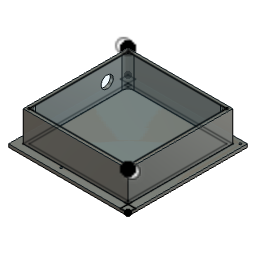
battery enclosure v1 (Autodesk Fusion 360 design; units mm, degrees)
Autodesk Fusion 360 part; units mm, degrees
sketch "Sketch1" plane through (0, 0, 0) normal (0, 1, 0) x (1, 0, 0)
  line L0 (0, 0) -> (196, 0)
  line L1 (196, 0) -> (196, 196)
  line L2 (196, 196) -> (0, 196)
  line L3 (0, 196) -> (0, 0)
  dimension "d1" = 196
  dimension "d2" = 196
  constraint horizontal L0
  constraint vertical L1
  constraint horizontal L2
  constraint vertical L3
  constraint coincident L0.start L3.end
  measures "d1" distance of L0.start L0.end
  measures "d2" distance of L0.start L2.end
extrude "Extrude1" add sketch "Sketch1" along normal blind 5
sketch "Sketch2" plane through (0, 5, 0) normal (0, 1, 0) x (-1, 0, 0)
  line L0 (0, -196) -> (0, 0)
  line L1 (0, 0) -> (-196, 0)
  line L2 (-196, 0) -> (-196, -196)
  line L3 (-196, -196) -> (0, -196)
  line L4 (0, 0) -> (-77, 0)
  line L5 (-77, 0) -> (-77, -9)
  line L6 (-77, -9) -> (0, -9)
  line L7 (0, -9) -> (0, 0)
  line L8 (0, -196) -> (-5.6569, -190.3431)
  line L9 (0, -196) -> (8, -196) construction
  line L10 (-196, -196) -> (-190.3431, -190.3431)
  line L11 (-196, -196) -> (-188, -196) construction
  dimension "d5" = 77
  dimension "d6" = 9
  dimension "d7" = 135
  dimension "d8" = 8
  dimension "d9" = 45
  dimension "d10" = 8
  constraint horizontal L4
  constraint vertical L5
  constraint horizontal L6
  constraint vertical L7
  constraint coincident L0.end L1.start
  constraint horizontal L9
  constraint coincident L0.start L3.end
  constraint horizontal L11
  constraint coincident L2.end L3.start
  measures "d5" distance of L0.end L4.end
  measures "d6" distance of L0.end L6.end
  measures "d7" angle of L8 L9
  measures "d8" distance of L0.start L8.end
  measures "d9" angle of L10 L11
  measures "d10" distance of L2.end L10.end
hole "Hole1" at (5.6569, 5, -190.3431) at (190.3431, 5, -190.3431) direction (0, -1, 0) diameter 3.5 depth 10 tip angle 180
hole "Hole2" at (77, 5, -9) direction (0, -1, 0) diameter 3.5 depth 10 tip angle 180
sketch "Sketch3" plane through (0, 5, 0) normal (0, 1, 0) x (-1, 0, 0)
  circle A0 centre (-77, -9) radius 1.75
  circle A1 centre (-5.6569, -190.3431) radius 1.75
  circle A2 centre (-190.3431, -190.3431) radius 1.75
  line L0 (0, -196) -> (0, 0)
  line L1 (0, 0) -> (-196, 0)
  line L2 (-196, 0) -> (-196, -196)
  line L3 (-196, -196) -> (0, -196)
  line L4 (0, -196) -> (-12, -196)
  line L5 (-12, -196) -> (-12, -184)
  line L6 (-12, -184) -> (0, -184)
  line L7 (0, -184) -> (0, -196)
  line L8 (-196, 0) -> (-184, 0)
  line L9 (-184, 0) -> (-184, -12)
  line L10 (-184, -12) -> (-196, -12)
  line L11 (-196, -12) -> (-196, 0)
  line L12 (-12, -184) -> (-184, -184)
  line L13 (-184, -184) -> (-184, -12)
  line L14 (-184, -12) -> (-12, -12)
  line L15 (-12, -12) -> (-12, -184)
  line L16 (-12, -184) -> (-17, -184)
  line L17 (-17, -184) -> (-17, -179)
  line L18 (-17, -179) -> (-12, -179)
  line L19 (-12, -179) -> (-12, -184)
  line L20 (-184, -12) -> (-179, -12)
  line L21 (-179, -12) -> (-179, -17)
  line L22 (-179, -17) -> (-184, -17)
  line L23 (-184, -17) -> (-184, -12)
  line L24 (-17, -179) -> (-179, -179)
  line L25 (-179, -179) -> (-179, -17)
  line L26 (-179, -17) -> (-17, -17)
  line L27 (-17, -17) -> (-17, -179)
  dimension "d17" = 12
  dimension "d18" = 12
  dimension "d19" = 12
  dimension "d20" = 12
  dimension "d21" = 5
  dimension "d22" = 5
  dimension "d23" = 5
  dimension "d24" = 5
  constraint horizontal L4
  constraint vertical L5
  constraint horizontal L6
  constraint vertical L7
  constraint coincident L0.start L3.end
  constraint horizontal L8
  constraint vertical L9
  constraint horizontal L10
  constraint vertical L11
  constraint coincident L1.end L2.start
  constraint horizontal L12
  constraint vertical L13
  constraint horizontal L14
  constraint vertical L15
  constraint horizontal L16
  constraint vertical L17
  constraint horizontal L18
  constraint vertical L19
  constraint horizontal L20
  constraint vertical L21
  constraint horizontal L22
  constraint vertical L23
  constraint horizontal L24
  constraint vertical L25
  constraint horizontal L26
  constraint vertical L27
  measures "d17" distance of L0.start L4.end
  measures "d18" distance of L0.start L6.end
  measures "d19" distance of L1.end L8.end
  measures "d20" distance of L1.end L10.end
  measures "d21" distance of L5.end L16.end
  measures "d22" distance of L5.end L18.end
  measures "d23" distance of L9.end L20.end
  measures "d24" distance of L9.end L22.end
extrude "Extrude2" add sketch "Sketch3" along normal blind 50 contours L12 L15 L16 L17 L18 L19 | L12 L13 L17 L22 L24 L25 | L14 L15 L18 L21 L26 L27 | L13 L14 L20 L21 L22 L23
fillet "Fillet1" radius 10 1 edges at (17, 30, -179)
fillet "Fillet2" radius 10 1 edges at (179, 30, -179)
fillet "Fillet3" radius 10 1 edges at (179, 30, -17)
fillet "Fillet4" radius 10 1 edges at (17, 30, -17)
sketch "Sketch4" plane through (0, 55, 0) normal (0, 1, 0) x (-1, 0, 0)
  line L0 (-169, -17) -> (-27, -17)
  arc A0 (-17, -27) -> (-27, -17) centre (-27, -27) ccw
  line L1 (-17, -27) -> (-17, -169)
  arc A1 (-27, -179) -> (-17, -169) centre (-27, -169) ccw
  line L2 (-27, -179) -> (-169, -179)
  arc A2 (-179, -169) -> (-169, -179) centre (-169, -169) ccw
  line L3 (-179, -169) -> (-179, -27)
  arc A3 (-169, -17) -> (-179, -27) centre (-169, -27) ccw
  line L4 (-184, -12) -> (-184, -184)
  line L5 (-184, -184) -> (-12, -184)
  line L6 (-12, -184) -> (-12, -12)
  line L7 (-12, -12) -> (-184, -12)
  line L8 (-12, -184) -> (-16.9497, -179.0503)
  line L9 (-12, -184) -> (-5, -184) construction
  line L10 (-184, -12) -> (-179.0503, -16.9497)
  line L11 (-184, -12) -> (-191, -12) construction
  line L12 (-16.9497, -179.0503) -> (-179.0503, -179.0503)
  line L13 (-179.0503, -179.0503) -> (-179.0503, -16.9497)
  line L14 (-179.0503, -16.9497) -> (-16.9497, -16.9497)
  line L15 (-16.9497, -16.9497) -> (-16.9497, -179.0503)
  dimension "d35" = 135
  dimension "d36" = 7
  dimension "d37" = 135
  dimension "d38" = 7
  constraint horizontal L9
  constraint coincident L5.end L6.start
  constraint horizontal L11
  constraint coincident L4.start L7.end
  constraint horizontal L12
  constraint vertical L13
  constraint horizontal L14
  constraint vertical L15
  measures "d35" angle of L8 L9
  measures "d36" distance of L5.end L8.end
  measures "d37" angle of L10 L11
  measures "d38" distance of L4.start L10.end
hole "Hole3" at (16.9497, 55, -179.0503) direction (0, -1, 0) diameter 4.7 depth 4.3 tip angle 180
hole "Hole4" at (179.0503, 55, -179.0503) at (179.0503, 55, -16.9497) at (16.9497, 55, -16.9497) direction (0, -1, 0) diameter 4.7 depth 4.3 tip angle 180
hole "Hole5" at (12, 31.2423, -140.892) direction (1, 0, 0) diameter 4.7 depth 4.3 tip angle 180
hole "Hole6" at (12, 29.1387, -144.8388) direction (1, 0, 0) diameter 20 depth 4.3 tip angle 180
extrude "Extrude3" cut 1 faces at (16.3, 29.6025, -145.519) along direction (1, 0, 0) blind 105
